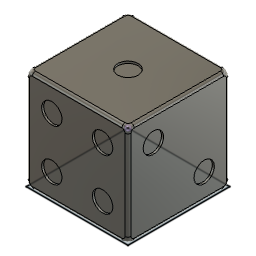
MMEZP_Kosticka v1 (Autodesk Fusion 360 design; units mm, degrees)
Autodesk Fusion 360 part; units mm, degrees
sketch "Sketch1" plane through (0, 0, 0) normal (0, 1, 0) x (1, 0, 0)
  line L0 (0, 0) -> (10, 0)
  line L1 (10, 0) -> (10, -10)
  line L2 (10, -10) -> (0, -10)
  line L3 (0, -10) -> (0, 0)
  dimension "d1" = 10
  dimension "d2" = 10
  constraint horizontal L0
  constraint vertical L1
  constraint horizontal L2
  constraint vertical L3
  constraint coincident L0.start L3.end
  measures "d1" distance of L0.start L0.end
  measures "d2" distance of L0.start L2.end
extrude "Extrude1" add sketch "Sketch1" along normal blind 10
sketch "Sketch2" plane through (0, 10, 0) normal (0, 1, 0) x (-1, 0, 0)
  line L0 (0, 10) -> (-10, 10)
  line L1 (-10, 10) -> (-10, 0)
  line L2 (-10, 0) -> (0, 0)
  line L3 (0, 0) -> (0, 10)
  circle A0 centre (-5, 5) radius 1
  dimension "d5" = 2
  dimension "d24" = 5
  dimension "d25" = 5
  measures "d5" diameter of A0
  measures "d24" distance of L3 A0.centre
  measures "d25" distance of L2 A0.centre
sketch "Sketch3" plane through (0, 0, 0) normal (0, -1, 0) x (1, 0, 0)
  line L0 (10, 10) -> (0, 10)
  line L1 (0, 10) -> (0, 0)
  line L2 (0, 0) -> (10, 0)
  line L3 (10, 0) -> (10, 10)
  circle A0 centre (3, 8) radius 1
  circle A1 centre (3, 5) radius 1
  circle A2 centre (3, 2) radius 1
  circle A3 centre (7, 8) radius 1
  circle A4 centre (7, 5) radius 1
  circle A5 centre (7, 2) radius 1
  dimension "d6" = 2
  dimension "d7" = 2
  dimension "d8" = 2
  dimension "d9" = 2
  dimension "d10" = 2
  dimension "d11" = 2
  dimension "d12" = 3
  dimension "d13" = 3
  dimension "d14" = 3
  dimension "d15" = 3
  dimension "d16" = 3
  dimension "d17" = 3
  dimension "d18" = 3
  dimension "d19" = 3
  dimension "d20" = 2
  dimension "d21" = 2
  dimension "d22" = 3
  dimension "d23" = 3
  measures "d6" diameter of A0
  measures "d7" diameter of A1
  measures "d8" diameter of A2
  measures "d9" diameter of A3
  measures "d10" diameter of A4
  measures "d11" diameter of A5
  measures "d12" distance of L3 A3.centre
  measures "d13" distance of L1 A0.centre
  measures "d14" distance of L1 A1.centre
  measures "d15" distance of L3 A4.centre
  measures "d16" distance of L3 A5.centre
  measures "d17" distance of L1 A2.centre
  measures "d18" distance of A0.centre A1.centre
  measures "d19" distance of A1.centre A2.centre
  measures "d20" distance of L0 A0.centre
  measures "d21" distance of L0 A3.centre
  measures "d22" distance of A3.centre A4.centre
  measures "d23" distance of A4.centre A5.centre
sketch "Sketch4" plane through (0, 0, 0) normal (-1, 0, 0) x (0, 0, 1)
  line L0 (0, 0) -> (10, 0)
  line L1 (10, 0) -> (10, 10)
  line L2 (10, 10) -> (0, 10)
  line L3 (0, 10) -> (0, 0)
  circle A0 centre (7.5, 2.5) radius 1
  circle A1 centre (5, 5) radius 1
  circle A2 centre (2.5, 7.5) radius 1
  circle A3 centre (2.5, 2.5) radius 1
  circle A4 centre (7.5, 7.5) radius 1
  line L4 (10, 0) -> (0, 0)
  line L5 (0, 10) -> (10, 10)
  dimension "d26" = 2
  dimension "d27" = 2
  dimension "d28" = 2
  dimension "d29" = 2
  dimension "d30" = 2
  dimension "d31" = 2.5
  dimension "d32" = 2.5
  dimension "d33" = 2.5
  dimension "d34" = 2.5
  dimension "d35" = 2.5
  dimension "d36" = 2.5
  dimension "d37" = 2.5
  dimension "d38" = 2.5
  dimension "d39" = 5
  dimension "d40" = 5
  measures "d26" diameter of A0
  measures "d27" diameter of A1
  measures "d28" diameter of A2
  measures "d29" diameter of A3
  measures "d30" diameter of A4
  measures "d31" distance of L3 A2.centre
  measures "d32" distance of L3 A3.centre
  measures "d33" distance of L1 A0.centre
  measures "d34" distance of L1 A4.centre
  measures "d35" distance of A3.centre L4
  measures "d36" distance of A2.centre L5
  measures "d37" distance of A4.centre L5
  measures "d38" distance of A0.centre L4
  measures "d39" distance of L3 A1.centre
  measures "d40" distance of A1.centre L4
sketch "Sketch5" plane through (0, 0, 0) normal (0, 0, -1) x (-1, 0, 0)
  line L0 (-10, 0) -> (0, 0)
  line L1 (0, 0) -> (0, 10)
  line L2 (0, 10) -> (-10, 10)
  line L3 (-10, 10) -> (-10, 0)
  circle A0 centre (-5, 5) radius 1
  circle A1 centre (-7.5, 2.5) radius 1
  circle A2 centre (-2.5, 7.5) radius 1
  line L4 (0, 10) -> (0, 0)
  line L5 (-10, 10) -> (0, 10)
  line L6 (0, 0) -> (-10, 0)
  dimension "d41" = 2
  dimension "d42" = 2
  dimension "d43" = 2
  dimension "d44" = 2.5
  dimension "d45" = 2.5
  dimension "d46" = 2.5
  dimension "d47" = 2.5
  dimension "d48" = 5
  dimension "d49" = 5
  measures "d41" diameter of A0
  measures "d42" diameter of A1
  measures "d43" diameter of A2
  measures "d44" distance of A2.centre L4
  measures "d45" distance of A2.centre L5
  measures "d46" distance of L3 A1.centre
  measures "d47" distance of A1.centre L6
  measures "d48" distance of L3 A0.centre
  measures "d49" distance of A0.centre L6
sketch "Sketch6" plane through (10, 0, 0) normal (1, 0, 0) x (0, 0, -1)
  line L0 (-10, 0) -> (0, 0)
  line L1 (0, 0) -> (0, 10)
  line L2 (0, 10) -> (-10, 10)
  line L3 (-10, 10) -> (-10, 0)
  circle A0 centre (-2.5, 2.5) radius 1
  circle A1 centre (-7.5, 7.5) radius 1
  line L4 (0, 0) -> (-10, 0)
  line L5 (-10, 10) -> (0, 10)
  dimension "d50" = 2
  dimension "d51" = 2
  dimension "d52" = 2.5
  dimension "d53" = 2.5
  dimension "d54" = 2.5
  dimension "d55" = 2.5
  measures "d50" diameter of A0
  measures "d51" diameter of A1
  measures "d52" distance of L1 A0.centre
  measures "d53" distance of A0.centre L4
  measures "d54" distance of L3 A1.centre
  measures "d55" distance of A1.centre L5
sketch "Sketch7" plane through (0, 0, 10) normal (0, 0, 1) x (1, 0, 0)
  line L0 (0, 0) -> (10, 0)
  line L1 (10, 0) -> (10, 10)
  line L2 (10, 10) -> (0, 10)
  line L3 (0, 10) -> (0, 0)
  circle A0 centre (7.5, 2.5) radius 1
  circle A1 centre (2.5, 7.5) radius 1
  circle A2 centre (2.5, 2.5) radius 1
  circle A3 centre (7.5, 7.5) radius 1
  line L4 (10, 0) -> (0, 0)
  line L5 (0, 0) -> (0, 10)
  line L6 (10, 10) -> (10, 0)
  dimension "d56" = 2
  dimension "d57" = 2
  dimension "d58" = 2
  dimension "d59" = 2
  dimension "d60" = 2.5
  dimension "d61" = 2.5
  dimension "d62" = 2.5
  dimension "d63" = 2.5
  dimension "d64" = 2.5
  dimension "d65" = 2.5
  dimension "d66" = 2.5
  dimension "d67" = 2.5
  measures "d56" diameter of A0
  measures "d57" diameter of A1
  measures "d58" diameter of A2
  measures "d59" diameter of A3
  measures "d60" distance of L3 A2.centre
  measures "d61" distance of A2.centre L4
  measures "d62" distance of A1.centre L5
  measures "d63" distance of L2 A1.centre
  measures "d64" distance of A0.centre L6
  measures "d65" distance of A0.centre L4
  measures "d66" distance of A3.centre L6
  measures "d67" distance of L2 A3.centre
extrude "Extrude2" cut sketch "Sketch3" against normal blind 0.2 contours A0 | A1 | A2 | A3 | A4 | A5
extrude "Extrude3" cut sketch "Sketch7" against normal blind 0.2 contours A0 | A1 | A2 | A3
extrude "Extrude4" cut sketch "Sketch4" against normal blind 0.2 contours A0 | A1 | A2 | A3 | A4
extrude "Extrude5" cut sketch "Sketch6" against normal blind 0.2 contours A0 | A1
extrude "Extrude6" cut sketch "Sketch5" against normal blind 0.2 contours A0 | A1 | A2
extrude "Extrude7" cut sketch "Sketch2" against normal blind 0.2 contours A0
fillet "Fillet1" radius 0.3 12 edges at (0, 0, 5) (5, 0, 0) (0, 5, 0) (10, 0, 5) (10, 5, 0) (5, 10, 0) (10, 10, 5) (10, 5, 10) (5, 0, 10) (0, 5, 10) (0, 10, 5) (5, 10, 10)
